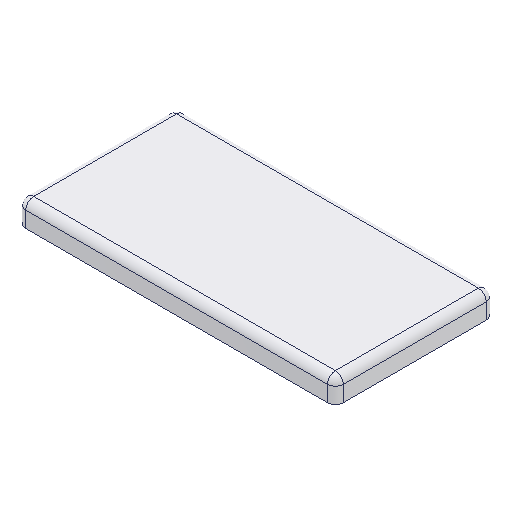
# Autodesk Inventor part: COTS_GENERIC_20x40_Alu_Extrusion_Endcap
Saved by Autodesk Inventor 2026.1 (Build 301233000, 233)
## iProperties
Created: 2017-05-23
Part Number: COTS_GENERIC_20x40_Alu_Extrusion_Endcap
Material: Ogólny
Document SubType Name: Modeling
Designer: Andrzej
Density: 1 g/cm^3
Appearance: PTFE
Mass: 2.37234 g
Surface Area: 19.0192 cm^2
Volume: 2.37234 cm^3
Author: Andrzej
Autodesk Inventor part; units mm, degrees
ref_plane "YZ Plane" through (0, 0, 0) normal (1, 0, 0) x (0, 1, 0)
ref_plane "XZ Plane" through (0, 0, 0) normal (0, 1, 0) x (-1, 0, 0)
ref_plane "XY Plane" through (0, 0, 0) normal (0, 0, 1) x (1, 0, 0)
sketch "Szkic1" plane through (0, 0, 0) normal (0, 0, 1) x (1, 0, 0)
  line L0 (-8.4451, 5.1519) -> (31.5549, 5.1519)
  line L1 (31.5549, 5.1519) -> (31.5549, -14.8481)
  line L2 (31.5549, -14.8481) -> (-8.4451, -14.8481)
  line L3 (-8.4451, -14.8481) -> (-8.4451, 5.1519)
  point P0 (0, 0)
  dimension "d0" = 40
  dimension "d1" = 20
  constraints: 8 end point, 2 parallel, 1 horizontal, 1 perpendicular
  measures "d0" distance of L1.end L2.end
  measures "d1" distance of L0.end L1.end
extrude "Wyciągnięcie proste1" add sketch "Szkic1" along normal blind 3
fillet "Zaokrąglenie1" radius 1 4 edges at (-8.4451, 5.1519, 1.5) (31.5549, 5.1519, 1.5) (31.5549, -14.8481, 1.5) (-8.4451, -14.8481, 1.5)
fillet "Zaokrąglenie2" radius 1 8 edges at (-8.1522, 4.859, 3) (-8.4451, -4.8481, 3) (-8.1522, -14.5552, 3) (11.5549, -14.8481, 3) (31.262, -14.5552, 3) (31.5549, -4.8481, 3) (31.262, 4.859, 3) (11.5549, 5.1519, 3)
